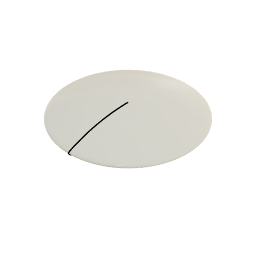
kamera-lidar-gnss v10 (Autodesk Fusion 360 archive; units mm, degrees)
design "Antenna"
Autodesk Fusion 360 part; units mm, degrees
sketch "antenna profile" plane through (0, 0, 0) normal (1, 0, 0) x (0, 1, 0)
  line L0 (0, 55.5) -> (0, 0)
  spline S0 degree 5 poles (-14.9144, 0) (-15.1986, 0) (-15.7331, 0.1601) (-16.4411, 0.8835) (-17.3417, 2.6008) (-19.257, 5.1416) (-21.0386, 6.927) (-22.1024, 8.041) (-23.9195, 9.5767) (-27.6306, 12.3835) (-32.1149, 15.2307) (-36.3626, 17.4398) (-39.8889, 18.971) (-42.5997, 20.0513) (-44.7474, 21.0551) (-47.2507, 22.1995) (-50.5943, 23.5558) (-54.5655, 25.1581) (-58.7737, 26.9955) (-62.7402, 29.0184) (-66.4348, 31.2125) (-69.908, 33.4457) (-72.712, 35.4368) (-74.3486, 36.9963) (-74.3085, 38.1824) (-72.3633, 39.478) (-68.9176, 40.998) (-64.5427, 42.7402) (-59.8013, 44.5945) (-54.755, 46.4647) (-49.1279, 48.2967) (-42.9246, 50.0271) (-36.1857, 51.6013) (-29.0488, 52.9679) (-21.681, 54.0822) (-14.2672, 54.9071) (-8.4331, 55.3128) (-4.1677, 55.466) (-1.38, 55.5) (0, 55.5) knots 0 0 0 0 0 0 0.028571 0.057143 0.085714 0.114286 0.142857 0.171429 0.2 0.228571 0.257143 0.285714 0.314286 0.342857 0.371429 0.4 0.428571 0.457143 0.485714 0.514286 0.542857 0.571429 0.6 0.628571 0.657143 0.685714 0.714286 0.742857 0.771429 0.8 0.828571 0.857143 0.885714 0.914286 0.942857 0.971429 1 1 1 1 1 1
  line L1 (-6.7465, 0) -> (-23.0822, 0)
  line L2 (-8.522, -7.6693) -> (-30.0208, 17.7018)
  line L3 (-10.6014, 0) -> (-42.251, 22.8292)
  line L4 (-35.5679, 16.868) -> (-53.4299, 25.0058)
  line L5 (-72.2398, 39.8804) -> (-46.5495, 49.5647)
  line L6 (-14.9866, 55.5) -> (14.9866, 55.5)
  line L7 (0, 0) -> (-14.9144, 0)
  line L8 (-47.055, 20.4473) -> (-78.5648, 37.8239)
  line L9 (-73.6324, 32.8325) -> (-74.5715, 41.9888)
  point P0 (-62.8099, 29.1356)
  point P1 (-26.4262, 11.4146)
  point P2 (-19.2714, 5.0163)
  point P3 (-44.4989, 20.9369)
  point P4 (-59.3947, 44.7226)
  point P5 (-74.102, 37.4107)
  dimension "d29" = 55.5
  constraint midpoint P2 L2
  constraint midpoint P3 L4
  constraint midpoint P1 L3
  constraint horizontal L7
  constraint midpoint S0.start L1
  constraint coincident L1.start L7
  constraint coincident L0.end L7.start
  constraint midpoint L0.start L6
  constraint midpoint P4 L5
  constraint vertical L0
  constraint midpoint P0 L8
  constraint coincident L3.start L1
  constraint coincident L3.start L7
  constraint midpoint P5 L9
  constraint horizontal L6
  measures "d29" distance of L0.start L7
sketch "Sketch8" plane through (0, 0, 0) normal (0, 0, 1) x (1, 0, 0)
revolve "Revolve1" add sketch "antenna profile" angle 360 about axis through (0, 0, 55.5) along (0, 0, -1) contours L0 S0 L1 L3 L7 | S0 L1 L2 L3 L7 | S0 L2 L3 | S0 L2
ref_plane "WorkPlane1" through (0, 0, 25) normal (0, 0, 1) x (1, 0, 0)
sketch "mounting" plane through (0, 0, 25) normal (0, 0, 1) x (1, 0, 0)
  circle A0 centre (0, 0) radius 25
  circle A1 centre (0, 0) radius 75
  line L0 (0, -75) -> (0, -25)
  line L1 (25, -0.0001) -> (75, -0.0001)
  line L2 (17.6777, -72.8869) -> (17.6777, -17.6777)
  line L3 (72.8869, -17.6777) -> (17.6777, -17.6777)
  line L4 (0, 0) -> (53.033, -53.033)
  dimension "d32" = 50
  dimension "d33" = 150
  constraint coincident A0.centre A1.centre
  constraint concentric A0 A1
  constraint coincident A1 L0.start
  constraint coincident A0 L0.end
  constraint vertical L0
  constraint coincident A0 L1.start
  constraint coincident A1 L1.end
  constraint coincident A1 L2.start
  constraint coincident A0 L2.end
  constraint vertical L2
  constraint coincident A1 L3.start
  constraint perpendicular L2 L3
  constraint coincident A1 L4.end
  constraint coincident L2.end L4
  constraint equal L2 L3
  constraint equal L0 L1
  constraint horizontal L1
  measures "d32" diameter of A0
  measures "d33" diameter of A1
extrude "Extrude3" cut sketch "mounting" against normal blind 40 contours A1 L2 L4 | A1 L3 L4
